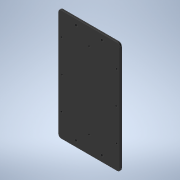
# Autodesk Inventor part: BatteryHolderBottom
Saved by Autodesk Inventor 2021 (Build 250183000, 183)
## iProperties
Created: 2021-02-16
Part Number: BatteryHolderBottom
Material: Generic
Document SubType Name: Modeling
Designer: Viktor
Density: 1 g/cm^3
Appearance: Default
Author: Viktor
Autodesk Inventor part; units mm, degrees
ref_plane "YZ Plane" through (0, 0, 0) normal (1, 0, 0) x (0, 1, 0)
ref_plane "XZ Plane" through (0, 0, 0) normal (0, 1, 0) x (-1, 0, 0)
ref_plane "XY Plane" through (0, 0, 0) normal (0, 0, 1) x (1, 0, 0)
sketch "Sketch1" plane through (0, 0, 0) normal (0, 0, 1) x (1, 0, 0)
  line L0 (-52.5, -95) -> (52.5, -95)
  line L1 (52.5, -95) -> (52.5, 95)
  line L2 (52.5, 95) -> (-52.5, 95)
  line L3 (-52.5, 95) -> (-52.5, -95)
  line L4 (-52.5, -95) -> (52.5, 95) construction
  line L5 (52.5, -95) -> (-52.5, 95) construction
  point P0 (0, 0)
  dimension "d0" = 190
  dimension "d1" = 105
  constraints: 12 end point, 2 midpoint, 2 parallel, 1 horizontal, 1 perpendicular
  measures "d0" distance of L2.end L0.start
  measures "d1" distance of L1.end L2.end
extrude "Extrusion1" add sketch "Sketch1" along normal blind 3
sketch "Sketch2" plane through (0, 0, 3) normal (0, 0, 1) x (1, 0, 0)
  circle A0 centre (-47, 55) radius 1.75
  line L0 (-52.5, 95) -> (-52.5, -95) construction
  line L1 (-73.5, 0) -> (73.5, 0) projected
  line L2 (0, 133) -> (0, -133) projected
  circle A1 centre (47, 55) radius 1.75
  circle A2 centre (-47, -55) radius 1.75
  circle A3 centre (47, -55) radius 1.75
  point P0 (0, 0)
  point P1 (52.5, 95)
  point P2 (52.5, -95)
  dimension "d6" = 47
  dimension "d7" = 3.5
  dimension "d8" = 55
  constraints: 5 symmetric about line, 4 centre point, 3 other
  measures "d6" horizontal distance of A0.centre point (0, 0)
  measures "d7" diameter of A0
  measures "d8" vertical distance of point (0, 0) A0.centre
extrude "Extrusion2" cut sketch "Sketch2" against normal blind 3
sketch "Sketch3" plane through (0, 0, 3) normal (0, 0, 1) x (1, 0, 0)
  circle A0 centre (-22, 85) radius 2.25
  line L0 (52.5, 95) -> (-52.5, 95) construction
  line L1 (0, 133) -> (0, -133) projected
  line L2 (-73.5, 0) -> (73.5, 0) projected
  circle A1 centre (22, 85) radius 2.25
  circle A2 centre (-22, -85) radius 2.25
  line L3 (52.5, -95) -> (-52.5, -95) construction
  circle A3 centre (22, -85) radius 2.25
  point P0 (0, 0)
  dimension "d11" = 10
  dimension "d12" = 4.5
  constraints: 5 symmetric about line, 4 centre point, 2 end point, 3 other
  measures "d11" distance from line of L0 A0.centre
  measures "d12" diameter of A0
extrude "Extrusion3" cut sketch "Sketch3" against normal blind 3
sketch "Sketch4" plane through (0, 0, 3) normal (0, 0, 1) x (1, 0, 0)
  line L0 (-40, -59) -> (40, -59) construction
  line L1 (40, -59) -> (40, 59) construction
  line L2 (40, 59) -> (-40, 59) construction
  line L3 (-40, 59) -> (-40, -59) construction
  line L4 (-40, -59) -> (40, 59) construction
  line L5 (40, -59) -> (-40, 59) construction
  line L6 (-73.5, 0) -> (73.5, 0) construction
  line L7 (0, -133) -> (0, 133) construction
  circle A0 centre (0, 65.25) radius 1.75
  circle A1 centre (-46.25, 0) radius 1.75
  circle A2 centre (0, -65.25) radius 1.75
  circle A3 centre (46.25, 0) radius 1.75
  line L8 (-52.5, 95) -> (-52.5, -95) projected
  circle A4 centre (-47, -55) radius 1.75 projected
  circle A5 centre (-47, 55) radius 1.75 projected
  point P0 (0, 0)
  dimension "d15" = 80
  dimension "d16" = 118
  dimension "d17" = 3.5
  dimension "d18" = 3.5
  dimension "d19" = 12.5
  dimension "d21" = 6.25
  dimension "d24" = 6.25
  dimension "d29" = 110
  constraints: 12 end point, 4 centre point, 2 midpoint, 2 parallel, 2 point on line, 2 symmetric about line, 1 horizontal, 1 perpendicular, 2 other
  measures "d15" distance of L1.end L2.end
  measures "d16" distance of L0.end L1.end
  measures "d17" diameter of A1
  measures "d18" diameter of A0
  measures "d19" distance between parallel lines of L3 L8
  measures "d21" distance from line of L2 A0.centre
  measures "d24" distance from line of L3 A1.centre
  measures "d29" distance of A4.centre A5.centre
extrude "Extrusion4" cut sketch "Sketch4" against normal blind 3 contours A0 | A1 | A2 | A3
fillet "Fillet1" radius 5 4 edges at (-52.5, -95, 1.5) (52.5, -95, 1.5) (52.5, 95, 1.5) (-52.5, 95, 1.5)
chamfer "Chamfer1" distance 0.5 angle 45 8 edges at (-52.5, 0, 3) (-51.0355, -93.5355, 3) (0, -95, 3) (51.0355, -93.5355, 3) (52.5, 0, 3) (51.0355, 93.5355, 3) (0, 95, 3) (-51.0355, 93.5355, 3)
equation "\"d18\" = d17"
equation "\"d21\" = d24"
equation "\"d24\" = 0.5 * d19"
body "Solid1"
